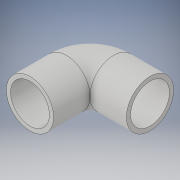
# Autodesk Inventor part: 90 Elbow 1 Inch
Saved by Autodesk Inventor 2018 (Build 220112000, 112)
## iProperties
Created: 2018-01-18
Part Number: 90 Elbow 1 Inch
Material: Generic
Document SubType Name: Modeling
Designer: owner
Density: 1 g/cm^3
Appearance: Default
Author: owner
Autodesk Inventor part; units mm, degrees
sketch "Sketch1" plane through (0, 0, 0) normal (0, 0, 1) x (1, 0, 0)
  circle A0 centre (0, 0) radius 20.3835
  dimension "d0" = 40.767
  constraints: 1 centre point, 1 coincident
  measures "d0" diameter of A0
extrude "Extrusion1" add sketch "Sketch1" against normal blind 31.4198
sketch "Sketch2" plane through (0, 0, -31.4198) normal (0, 0, -1) x (-1, 0, 0)
  circle A0 centre (0, 0) radius 20.3835 projected
  line L0 (-20.3835, 0) -> (-20.3835, 24.6473)
  constraints: 2 end point, 2 vertical, 1 horizontal alignment, 1 other
ref_plane "Work Plane1" through (20.3835, 0, -31.4198) normal (1, 0, 0) x (0, 1, 0)
sketch "Sketch3" plane through (20.3835, 0, -31.4198) normal (1, 0, 0) x (0, 1, 0)
  line L0 (-20.3835, 0) -> (20.3835, 0) projected
  line L1 (0, 0) -> (0, -20.3835)
  circle A0 centre (0, -20.3835) radius 20.3835
  point P0 (0, 31.4198)
  dimension "d4" = 20.3835
  constraints: 2 end point, 1 coincident, 1 midpoint, 1 vertical, 1 vertical alignment, 2 other
  measures "d4" distance of L1.start L1.end
extrude "Extrusion2" add sketch "Sketch3" along normal blind 31.4198
sketch "Sketch4" plane through (0, 0, 0) normal (0, 0, 1) x (1, 0, 0)
  circle A0 centre (0, 0) radius 16.7767
  dimension "d7" = 33.5534
  constraints: 1 centre point, 1 coincident
  measures "d7" diameter of A0
sketch "Sketch5" plane through (51.8033, 0, -51.8033) normal (1, 0, 0) x (0, 0, -1)
  circle A0 centre (0, 0) radius 16.7767
  point P0 (-51.8033, 0)
  dimension "d8" = 33.5534
  constraints: 1 centre point
  measures "d8" diameter of A0
ref_plane "Work Plane2" through (0, 0, -31.4198) normal (0, 0, -1) x (-1, 0, 0)
ref_plane "Work Plane3" through (20.3835, 0, -31.4198) normal (-1, 0, 0) x (0, 0, 1)
revolve "Revolution1" add sketch "Sketch2" angle 90 about axis through (20.3835, 0, -31.4198) along (0, -1, 0)
extrude "Extrusion3" cut sketch "Sketch4" against normal blind 31.75
sketch "Sketch6" plane through (0, 0, -31.4198) normal (0, 0, -1) x (-1, 0, 0)
  circle A0 centre (0, 0) radius 12.7
  line L0 (-20.3835, -28.5369) -> (-20.3835, 28.5369) projected
  dimension "d14" = 25.4
  constraints: 1 centre point, 1 coincident
  measures "d14" diameter of A0
revolve "Revolution2" cut sketch "Sketch6" angle 90 about axis through (20.3835, 0, -31.4198) along (0, -1, 0)
extrude "Extrusion4" cut sketch "Sketch5" against normal blind 31.75
body "Solid1"
